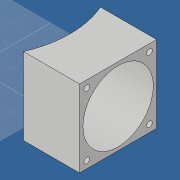
# Autodesk Inventor part: Bohrhilfe
Saved by Autodesk Inventor 2019 (Build 230136000, 136)
## iProperties
Created: 2020-07-30
Part Number: Bohrhilfe
Material: Generisch
Document SubType Name: Modeling
Designer: Stefan
Mass: 114.873 g
Surface Area: 385.116 cm^2
Volume: 114.873 cm^3
Density: 1 g/cm^3
Appearance: Vorgabe
Author: Stefan
Autodesk Inventor part; units mm, degrees
ref_plane "YZ Plane" through (0, 0, 0) normal (1, 0, 0) x (0, 1, 0)
ref_plane "XZ Plane" through (0, 0, 0) normal (0, 1, 0) x (-1, 0, 0)
ref_plane "XY Plane" through (0, 0, 0) normal (0, 0, 1) x (1, 0, 0)
sketch "Skizze1" plane through (0, 0, 0) normal (0, 1, 0) x (-1, 0, 0)
  circle A0 centre (0, 0) radius 100
  circle A1 centre (0, 0) radius 95.1
  line L0 (100, 0) -> (-150, 0) construction
  line L1 (-91.6515, 40) -> (-150, 40)
  line L2 (-150, 40) -> (-150, -40)
  line L3 (-150, -40) -> (-91.6515, -40)
  dimension "d0" = 200
  dimension "d1" = 4.9
  dimension "d2" = 150
  dimension "d3" = 80
  constraints: 8 end point, 3 point on circle, 2 centre point, 2 coincident, 2 horizontal, 2 perpendicular, 1 midpoint, 1 point on line
  measures "d0" diameter of A0
  measures "d1" radial gap between concentric circles of A0 A1
  measures "d2" distance of L0.end A0.centre
  measures "d3" distance between parallel lines of L3 L1
extrude "Extrusion1" add sketch "Skizze1" along normal mid plane 80 contours A0 L3 L2 L1
sketch "Skizze2" plane through (150, -40, -40) normal (1, 0, 0) x (0, 0, -1)
  circle A0 centre (-40, 40) radius 36.5
  line L0 (-72.5, 7.5) -> (-7.5, 7.5)
  line L1 (-7.5, 7.5) -> (-7.5, 72.5)
  line L2 (-7.5, 72.5) -> (-72.5, 72.5)
  line L3 (-72.5, 72.5) -> (-72.5, 7.5)
  line L4 (-72.5, 7.5) -> (-7.5, 72.5) construction
  line L5 (-7.5, 7.5) -> (-72.5, 72.5) construction
  circle A1 centre (-72.5, 72.5) radius 3
  circle A2 centre (-7.5, 72.5) radius 3
  circle A3 centre (-7.5, 7.5) radius 3
  circle A4 centre (-72.5, 7.5) radius 3
  point P0 (-40, 40)
  dimension "d6" = 73
  dimension "d9" = 65
  dimension "d10" = 6
  constraints: 12 end point, 5 centre point, 5 coincident, 3 equal radius, 2 midpoint, 2 parallel, 2 perpendicular, 1 horizontal
  measures "d6" diameter of A0
  measures "d9" distance of L1.end L2.end
  measures "d10" diameter of A1
extrude "Extrusion2" cut sketch "Skizze2" against normal through all contours A0 L1 | L1 A0 L0 L3 L2 | L2 A0 | A2 L2 L1 | L1 L2 A2 | A0 L0 | A3 L0 L1 | L1 L0 A3 | L3 A0 | A1 L3 L2 | L2 L3 A1 | A4 L3 L0 | L0 L3 A4
equation "\"d0\" = kg_diameter"
equation "\"d1\" = kg_thickness"
equation "\"d4\" = d3"
equation "\"d6\" = bore_diameter"
equation "\"kg_diameter\" = 200"
equation "\"kg_thickness\" = 4.9"
equation "\"ht_thickness\" = 1.9"
equation "\"case_thickness\" = 18"
equation "\"gap_fit\" = 0.1"
equation "\"gap_slide\" = 0.2"
equation "\"gap_air\" = 1"
equation "\"bore_diameter\" = 73"
